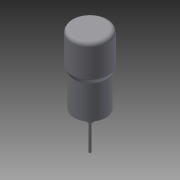
# Autodesk Inventor part: 1617evs
Saved by Autodesk Inventor 2014 (Build 180170000, 170)
## iProperties
Created: 2014-08-20
Part Number: 1617evs
Material: Generic
Document SubType Name: Modeling
Designer: Matthew
Density: 1 g/cm^3
Appearance: Default
Author: Matthew
Autodesk Inventor part; units mm, degrees
ref_plane "YZ Plane" through (0, 0, 0) normal (1, 0, 0) x (0, 1, 0)
ref_plane "XZ Plane" through (0, 0, 0) normal (0, 1, 0) x (-1, 0, 0)
ref_plane "XY Plane" through (0, 0, 0) normal (0, 0, 1) x (1, 0, 0)
sketch "Sketch1" plane through (0, 0, 0) normal (0, 1, 0) x (-1, 0, 0)
  circle A0 centre (0, 0) radius 50.8
  dimension "d0" = 101.6
  constraints: 1 centre point, 1 coincident
  measures "d0" diameter of A0
extrude "Extrusion1" add sketch "Sketch1" along normal blind 88.9
fillet "Fillet1" radius 10.16 1 edges at (50.8, 88.9, 0)
sketch "Sketch2" plane through (0, 0, 0) normal (0, -1, 0) x (1, 0, 0)
  circle A0 centre (0, 0) radius 50.8 projected
  circle A1 centre (0, 0) radius 44.45
  dimension "d4" = 88.9
  constraints: 1 centre point, 1 coincident
  measures "d4" diameter of A1
extrude "Extrusion2" add sketch "Sketch2" along normal blind 12.7 contours A1
loft "Loft1" add section 1 edges at (50.8, 0, 0) section 2 edges at (-44.45, -12.7, 0)
fillet "Fillet2" radius 5.08 1 edges at (50.8, 0, 0)
sketch "Sketch3" plane through (0, -12.7, 0) normal (0, -1, 0) x (1, 0, 0)
  circle A0 centre (0, 0) radius 44.45 projected
extrude "Extrusion3" add sketch "Sketch3" along normal blind 92.075
sketch "Sketch4" plane through (0, -104.775, 0) normal (0, -1, 0) x (1, 0, 0)
  circle A0 centre (0, 0) radius 44.45 projected
  circle A1 centre (0, 0) radius 9.525
  dimension "d14" = 19.05
  constraints: 1 centre point, 1 coincident
  measures "d14" diameter of A1
extrude "Extrusion4" add sketch "Sketch4" along normal blind 28.575 contours A1
sketch "Sketch5" plane through (0, -133.35, 0) normal (0, -1, 0) x (1, 0, 0)
  circle A0 centre (0, 0) radius 9.525 projected
  circle A1 centre (0, 0) radius 3.175
  dimension "d17" = 6.35
  constraints: 1 centre point, 1 coincident
  measures "d17" diameter of A1
extrude "Extrusion5" add sketch "Sketch5" along normal blind 88.9 contours A1
body "Solid1"
